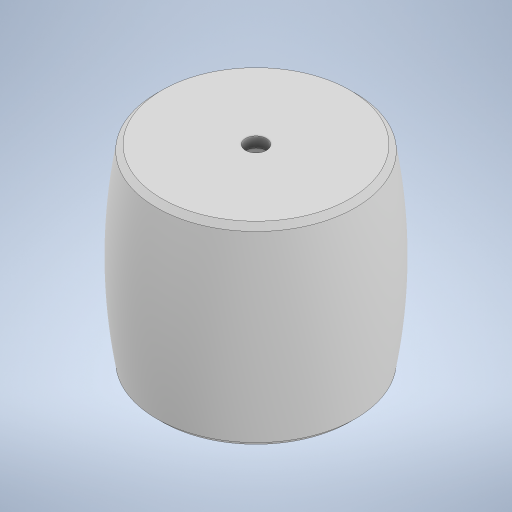
# Autodesk Inventor part: Part2
Saved by Autodesk Inventor 2024 (Build 280153000, 153)
## iProperties
Created: 2023-12-17
Part Number: Part2
Material: Generic
Document SubType Name: Modeling
Designer: SAHITYA
Density: 1 g/cm^3
Appearance: Default
Author: SAHITYA
Autodesk Inventor part; units mm, degrees
ref_plane "YZ Plane" through (0, 0, 0) normal (1, 0, 0) x (0, 1, 0)
ref_plane "XZ Plane" through (0, 0, 0) normal (0, 1, 0) x (-1, 0, 0)
ref_plane "XY Plane" through (0, 0, 0) normal (0, 0, 1) x (1, 0, 0)
sketch "Sketch1" plane through (0, 0, 0) normal (1, 0, 0) x (0, 1, 0)
  line L0 (7.6074, 5.6556) -> (7.6074, -12.3444)
  line L1 (7.6074, 5.6556) -> (-10.8926, 5.6556)
  line L2 (-10.8926, 5.6556) -> (-10.8926, -12.3444)
  line L3 (-10.8926, -12.3444) -> (7.6074, -12.3444)
  line L4 (7.6074, -3.3444) -> (7.6074, -12.3444)
  line L5 (7.1074, -12.8444) -> (-10.3926, -12.8444)
  line L6 (-10.8926, -12.3444) -> (-10.8926, -12.3444)
  line L7 (7.6074, -12.3444) -> (7.1074, -12.8444)
  line L8 (-10.8926, -12.3444) -> (-10.3926, -12.8444)
  arc A0 (-10.3926, -12.8444) -> (7.1074, -12.8444) centre (-1.6426, 37.3994) ccw
  line L9 (7.6074, -3.3444) -> (-10.8926, -3.3444)
  line L10 (-10.8926, 5.6556) -> (7.6074, 5.6556)
  line L11 (7.1074, 6.1556) -> (-10.3926, 6.1556)
  line L12 (-10.8926, 5.6556) -> (-10.8926, 5.6556)
  line L13 (7.6074, 5.6556) -> (7.1074, 6.1556)
  line L14 (-10.8926, 5.6556) -> (-10.3926, 6.1556)
  arc A1 (7.1074, 6.1556) -> (-10.3926, 6.1556) centre (-1.6426, -44.0882) ccw
  line L15 (-1.6426, -13.6006) -> (-1.6426, -3.3444) construction
  point P0 (0, 0)
  point P1 (7.6074, -12.8444)
  point P2 (-10.8926, -12.8444)
  point P3 (7.6074, 6.1556)
  point P4 (-10.8926, 6.1556)
  point P5 (-1.6426, 6.9118)
  dimension "d0" = 18
  dimension "d1" = 18.5
  dimension "d2" = 9.5
  dimension "d3" = 0.5
  dimension "d4" = 0.5
  dimension "d5" = 0.5
  dimension "d6" = 0.5
  dimension "d7" = 51
  dimension "d8" = 10.2562
  dimension "d9" = 20.5124
  constraints: 32 end point, 10 symmetric about line, 9 point on line, 6 point on circle, 4 perpendicular, 3 midpoint, 2 centre point, 1 horizontal, 1 vertical, 1 other
  measures "d0" distance of L0.start L0.end
  measures "d1" distance of L0.start L1.end
  measures "d2" distance of L4.start point (7.607, -12.844)
  measures "d3" distance of L4.end point (7.607, -12.844)
  measures "d4" distance of L5.start point (7.607, -12.844)
  measures "d5" distance of L6.start point (-10.893, -12.844)
  measures "d6" distance of L5.end point (-10.893, -12.844)
  measures "d7" radius of A0
  measures "d8" distance of L15.start L15.end
  measures "d9" distance of L15.start point (-1.643, 6.912)
revolve "Revolution1" add sketch "Sketch1" angle 360 about axis through (0, 7.6074, -3.3444) along (0, -1, 0) contours L0 L3 L2 L9 | L7 L5 L8 L3 | A0 L5
sketch "Sketch2" plane through (0, 7.6074, -3.3444) normal (0, 1, 0) x (1, 0, 0)
  circle A0 centre (0, 0) radius 1
  circle A1 centre (0, 0) radius 9.5 projected
  circle A2 centre (0, 0) radius 1.1
  point P0 (0, -3.3444)
  dimension "d11" = 2
  dimension "d12" = 2.2
  constraints: 2 centre point, 1 coincident
  measures "d11" diameter of A0
  measures "d12" diameter of A2
extrude "Extrusion1" cut sketch "Sketch2" against normal blind 1.2 contours A0 | A2
sketch "Sketch3" plane through (0, -10.8926, -3.3444) normal (0, -1, 0) x (1, 0, 0)
  circle A0 centre (0, 0) radius 1.1 projected
  circle A1 centre (0, 0) radius 1.1
  point P0 (0, 3.3444)
  constraints: 1 centre point, 1 coincident
extrude "Extrusion2" cut sketch "Sketch3" against normal blind 1.2
sketch "Sketch4" plane through (0, -10.8926, -3.3444) normal (0, -1, 0) x (1, 0, 0)
  circle A0 centre (0, 0) radius 1
  circle A1 centre (0, 0) radius 1.1
  point P0 (0, 3.3444)
  dimension "d17" = 2
  constraints: 2 centre point, 1 coincident
  measures "d17" diameter of A0
extrude "Extrusion3" add sketch "Sketch4" against normal blind 1.2
sketch "Sketch5" plane through (0, 7.6074, -3.3444) normal (0, 1, 0) x (1, 0, 0)
  circle A0 centre (0, 0) radius 1
  circle A1 centre (0, 0) radius 1.1
  point P0 (0, -3.3444)
  constraints: 2 centre point, 1 coincident
extrude "Extrusion4" add sketch "Sketch5" against normal blind 1.2
sketch "Sketch6" plane through (0, 6.4074, -3.3444) normal (0, 1, 0) x (1, 0, 0)
  circle A0 centre (0, 0) radius 1
  point P0 (0, -3.3444)
  constraints: 1 centre point
extrude "Extrusion5" add sketch "Sketch6" along normal blind 0.2
sketch "Sketch7" plane through (0, -9.6926, -3.3444) normal (0, -1, 0) x (1, 0, 0)
  circle A0 centre (0, 0) radius 1
  point P0 (0, 3.3444)
  constraints: 1 centre point
extrude "Extrusion6" add sketch "Sketch7" along normal blind 0.2
equation "\"d4\" = d3"
equation "\"d6\" = d5"
body "Solid1"
